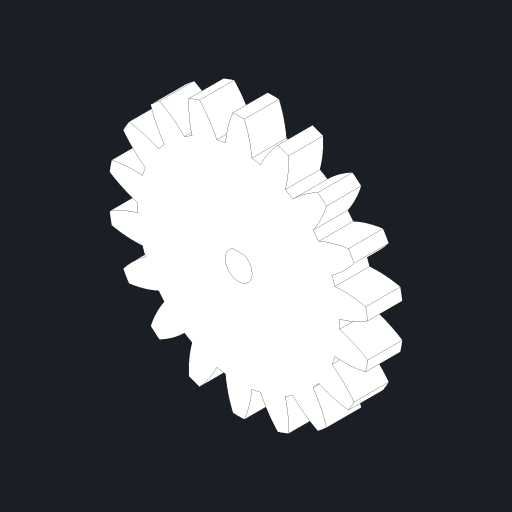
# Autodesk Inventor part: Spur Gear1
Saved by Autodesk Inventor 2024.3 (Build 283343000, 343)
## iProperties
CustomPartVersion: 1
Created: 2024-08-15
Part Number: Spur Gear1
Material: Steel
Document SubType Name: Modeling
Designer: Niler
Categories: <?xml version="1.0" encoding="UTF-16"?> <MemberInstance><Categories><FamilyTemplate><FamilyTemplateParameter ValueType="xs:double" Id="1" ObjectReferenceKey="da_z" ObjectType="kUserParameterObject"/><FamilyTemplateParameter ValueType="xs:double" Id="2" ObjectReferenceKey="da_b" ObjectType="kUserParameterObject"/><FamilyTemplateParameter ValueType="xs:double" Id="3" ObjectReferenceKey="da_beta" ObjectType="kUserParameterObject"/><FamilyTemplateParameter ValueType="xs:double" Id="4" ObjectReferenceKey="da_da" ObjectType="kUserParameterObject"/><FamilyTemplateParameter ValueType="xs:double" Id="5" ObjectReferenceKey="da_aw" ObjectType="kUserParameterObject"/><FamilyTemplateParameter ValueType="xs:string" Id="6" ObjectReferenceKey="EAIAABAAAACIAQAAAAAAAIAAAAAAAAAA" ObjectType="83910656" SubObjectId="SurfaceGeometry"/></FamilyTemplate><ParamToTemplateMap><ParamToTemplate CategoryParameter="//CategoryParameter[@InternalName='046C89C9-8512-4d59-83FE-43B91F4F132A']" TemplateParameter="1"/><ParamToTemplate CategoryParameter="//CategoryParameter[@InternalName='2552DF32-E462-4b46-AEBF-C6C7768E72AC']" TemplateParameter="2"/><ParamToTemplate CategoryParameter="//CategoryParameter[@InternalName='C9EE641D-15FC-4fae-A226-E94C4372FDD7']" TemplateParameter="3"/><ParamToTemplate><ParamToTemplate CategoryParameter="//CategoryParameter[@InternalName='00B6519A-459B-49c7-AD84-2E56D39A5744']" ConstantValue="0.000000"/></ParamToTemplate><ParamToTemplate><ParamToTemplate CategoryParameter="//CategoryParameter[@InternalName='04B31F0E-C7A6-4894-AA32-9629BEFACF47']" ConstantValue="1.000000"/></ParamToTemplate><ParamToTemplate><ParamToTemplate CategoryParameter="//CategoryParameter[@InternalName='43CBEC2E-7847-49e7-A936-2F7889FCB2D9']" ConstantValue="0.250000"/></ParamToTemplate><ParamToTemplate><ParamToTemplate CategoryParameter="//CategoryParameter[@InternalName='B1EFC894-105D-4ebd-86BF-FA20ED196853']" ConstantValue="0.350000"/></ParamToTemplate><ParamToTemplate><ParamToTemplate CategoryParameter="//CategoryParameter[@InternalName='51175063-3D10-4879-93E8-6246FE8B403D']" ConstantValue="2060000000.000000"/></ParamToTemplate><ParamToTemplate><ParamToTemplate CategoryParameter="//CategoryParameter[@InternalName='A3A52E27-4454-46a9-B0BD-C932399B70AF']" ConstantValue="0.300000"/></ParamToTemplate><ParamToTemplate><ParamToTemplate CategoryParameter="//CategoryParameter[@InternalName='91B76062-C214-41d9-B1B9-14D2AB99603D']" ConstantValue="0.300000"/></ParamToTemplate><ParamToTemplate><ParamToTemplate CategoryParameter="//CategoryParameter[@InternalName='374E806E-8B8A-4dda-A9AA-1039D6500AD2']" ConstantValue="3.333333"/></ParamToTemplate><ParamToTemplate><ParamToTemplate CategoryParameter="//CategoryParameter[@InternalName='2D373A89-B862-43d6-8D0B-0CBF12AB9F6C']" ConstantValue="0.349066"/></ParamToTemplate><ParamToTemplate CategoryParameter="//CategoryParameter[@InternalName='37777632-D6A2-4fac-9D53-DB8ACD95C989']" TemplateParameter="4"/><ParamToTemplate CategoryParameter="//CategoryParameter[@InternalName='FD1017F1-B727-4f7e-9707-0F86F1FF9423']" TemplateParameter="5"/><ParamToTemplate><ParamToTemplate CategoryParameter="//CategoryParameter[@InternalName='9E1B4470-B2D3-4ff1-B813-535BB4CDF51A']" ConstantValue="3520000.000000"/></ParamToTemplate><ParamToTemplate><ParamToTemplate CategoryParameter="//CategoryParameter[@InternalName='F8452263-BFF6-458c-9FB1-07C4B99E95CD']" ConstantValue="11400000.000000"/></ParamToTemplate><ParamToTemplate><ParamToTemplate CategoryParameter="//CategoryParameter[@InternalName='3E3BB259-FD49-497f-8171-6EBC954A3479']" ConstantValue="2.000000"/></ParamToTemplate><ParamToTemplate CategoryParameter="//CategoryParameter[@InternalName='27C3BAF2-7550-4e4b-AE2C-0DB134B7D9B7']" TemplateParameter="6"/></ParamToTemplateMap><Category DisplayName="Gear" InternalName="DC85795E-93AB-48d5-8EEE-5A27447B64BD" Mnemonic="Gear"><CategoryParameter DisplayName="z" InternalName="046C89C9-8512-4d59-83FE-43B91F4F132A" Mnemonic="z"/><CategoryParameter DisplayName="b" InternalName="2552DF32-E462-4b46-AEBF-C6C7768E72AC" Mnemonic="b"/><CategoryParameter DisplayName="||b|" InternalName="C9EE641D-15FC-4fae-A226-E94C4372FDD7" Mnemonic="beta"/><CategoryParameter DisplayName="x" InternalName="00B6519A-459B-49c7-AD84-2E56D39A5744" Mnemonic="x"/><CategoryParameter DisplayName="a*" InternalName="04B31F0E-C7A6-4894-AA32-9629BEFACF47" Mnemonic="a"/><CategoryParameter DisplayName="c*" InternalName="43CBEC2E-7847-49e7-A936-2F7889FCB2D9" Mnemonic="c"/><CategoryParameter DisplayName="r|.f|*" InternalName="B1EFC894-105D-4ebd-86BF-FA20ED196853" Mnemonic="rf"/><CategoryParameter DisplayName="E" InternalName="51175063-3D10-4879-93E8-6246FE8B403D" Mnemonic="E"/><CategoryParameter DisplayName="||m|" InternalName="A3A52E27-4454-46a9-B0BD-C932399B70AF" Mnemonic="mi"/><Category DisplayName="SpurGear" InternalName="26C5A22E-A91E-4dfd-A3B3-23CCAFAE1764" Mnemonic="SpurGear"><CategoryParameter DisplayName="m" InternalName="91B76062-C214-41d9-B1B9-14D2AB99603D" Mnemonic="m"/><CategoryParameter DisplayName="P" InternalName="374E806E-8B8A-4dda-A9AA-1039D6500AD2" Mnemonic="PP"/><CategoryParameter DisplayName="||a|" InternalName="2D373A89-B862-43d6-8D0B-0CBF12AB9F6C" Mnemonic="alpha"/><CategoryParameter DisplayName="d|.a|" InternalName="37777632-D6A2-4fac-9D53-DB8ACD95C989" Mnemonic="da"/><CategoryParameter DisplayName="a|.w|" InternalName="FD1017F1-B727-4f7e-9707-0F86F1FF9423" Mnemonic="aw"/><CategoryParameter DisplayName="||s||.Flim|" InternalName="9E1B4470-B2D3-4ff1-B813-535BB4CDF51A" Mnemonic="sFlim"/><CategoryParameter DisplayName="||s||.Hlim|" InternalName="F8452263-BFF6-458c-9FB1-07C4B99E95CD" Mnemonic="sHlim"/><CategoryParameter DisplayName="type" InternalName="3E3BB259-FD49-497f-8171-6EBC954A3479" Mnemonic="type"/><CategoryParameter DisplayName="PitchDiameter" InternalName="27C3BAF2-7550-4e4b-AE2C-0DB134B7D9B7" Mnemonic="IDS_PITCHDIAM"/></Category></Category></Categories></MemberInstance>
Density: 1 g/cm^3
Appearance: Steel
Author: Niler
Autodesk Inventor part; units mm, degrees
sketch "Sketch1" plane through (0, 0, 0) normal (0, 0, 1) x (1, 0, 0)
  circle A0 centre (0, 0) radius 30
  dimension "d0" = 60
  constraints: 1 centre point
  measures "d0" diameter of A0
extrude "Extrusion1" add sketch "Sketch1" along normal blind 8
ref_plane "Work Plane2" through (0, 0, 4) normal (0, 0, 1) x (1, 0, 0)
sketch "Sketch2" plane through (0, 0, 0) normal (0, 0, -1) x (-1, 0, 0)
  circle A0 centre (0, 0) radius 30 projected
  circle A1 centre (0, 0) radius 27
  dimension "d3" = 54
  constraints: 1 centre point, 1 coincident
  measures "d3" diameter of A1
surface extrude "Pitch Diameter" sketch "Sketch2" against normal through all shown no curves A1
ref_plane "Work Plane8" through (0, 0, 0) normal (0.9848078, 0.1736482, 0) x (0, 0, 1)
ref_plane "Work Plane9" through (0, 0, 0) normal (1, 0, 0) x (0, 1, 0)
spur gear teeth "Spur Gear" teeth 18 pitch diameter 54 tip diameter 60 root diameter 46.5 face width 8 start plane through (0, 0, 0) normal (0, 0, -1) x (-1, 0, 0)
sketch "Sketch3" plane through (0, 0, 0) normal (0, 0, -1) x (-1, 0, 0)
  circle A0 centre (0, 0) radius 3.1
  arc A1 (10.7357, 20.623) -> (11.4805, 27.7164) centre (-12.0166, 26.5979) ccw projected
  arc A2 (11.4805, 27.7164) -> (9.0212, 28.6115) centre (0, 0) ccw projected
  arc A3 (9.0212, 28.6115) -> (5.0322, 22.6989) centre (26.3021, 12.6511) ccw projected
  arc A4 (5.0322, 22.6989) -> (3.0347, 23.0511) centre (0, 0) ccw projected
  arc A5 (3.0347, 23.0511) -> (1.3086, 29.9714) centre (-20.389, 20.8839) ccw projected
  arc A6 (1.3086, 29.9714) -> (-1.3086, 29.9714) centre (0, 0) ccw projected
  arc A7 (-1.3086, 29.9714) -> (-3.0347, 23.0511) centre (20.389, 20.8839) ccw projected
  arc A8 (-3.0347, 23.0511) -> (-5.0322, 22.6989) centre (0, 0) ccw projected
  arc A9 (-5.0322, 22.6989) -> (-9.0212, 28.6115) centre (-26.3021, 12.6511) ccw projected
  arc A10 (-9.0212, 28.6115) -> (-11.4805, 27.7164) centre (0, 0) ccw projected
  arc A11 (-11.4805, 27.7164) -> (-10.7357, 20.623) centre (12.0166, 26.5979) ccw projected
  arc A12 (-10.7357, 20.623) -> (-12.4922, 19.6089) centre (0, 0) ccw projected
  arc A13 (-12.4922, 19.6089) -> (-18.2628, 23.8006) centre (-29.0428, 2.8923) ccw projected
  arc A14 (-18.2628, 23.8006) -> (-20.2677, 22.1183) centre (0, 0) ccw projected
  arc A15 (-20.2677, 22.1183) -> (-17.1417, 15.7075) centre (2.1949, 29.1038) ccw projected
  arc A16 (-17.1417, 15.7075) -> (-18.4455, 14.1537) centre (0, 0) ccw projected
  arc A17 (-18.4455, 14.1537) -> (-25.3017, 16.119) centre (-28.2805, -7.2154) ccw projected
  arc A18 (-25.3017, 16.119) -> (-26.6103, 13.8525) centre (0, 0) ccw projected
  arc A19 (-26.6103, 13.8525) -> (-21.4802, 8.8974) centre (-7.8916, 28.0993) ccw projected
  arc A20 (-21.4802, 8.8974) -> (-22.1739, 6.9914) centre (0, 0) ccw projected
  arc A21 (-22.1739, 6.9914) -> (-29.2889, 6.4932) centre (-24.1072, -16.4527) ccw projected
  arc A22 (-29.2889, 6.4932) -> (-29.7433, 3.9158) centre (0, 0) ccw projected
  arc A23 (-29.7433, 3.9158) -> (-23.2279, 1.0142) centre (-17.0262, 23.7057) ccw projected
  arc A24 (-23.2279, 1.0142) -> (-23.2279, -1.0142) centre (0, 0) ccw projected
  arc A25 (-23.2279, -1.0142) -> (-29.7433, -3.9158) centre (-17.0262, -23.7057) ccw projected
  arc A26 (-29.7433, -3.9158) -> (-29.2889, -6.4932) centre (0, 0) ccw projected
  arc A27 (-29.2889, -6.4932) -> (-22.1739, -6.9914) centre (-24.1072, 16.4527) ccw projected
  arc A28 (-22.1739, -6.9914) -> (-21.4802, -8.8974) centre (0, 0) ccw projected
  arc A29 (-21.4802, -8.8974) -> (-26.6103, -13.8525) centre (-7.8916, -28.0993) ccw projected
  arc A30 (-26.6103, -13.8525) -> (-25.3017, -16.119) centre (0, 0) ccw projected
  arc A31 (-25.3017, -16.119) -> (-18.4455, -14.1537) centre (-28.2805, 7.2154) ccw projected
  arc A32 (-18.4455, -14.1537) -> (-17.1417, -15.7075) centre (0, 0) ccw projected
  arc A33 (-17.1417, -15.7075) -> (-20.2677, -22.1183) centre (2.1949, -29.1038) ccw projected
  arc A34 (-20.2677, -22.1183) -> (-18.2628, -23.8006) centre (0, 0) ccw projected
  arc A35 (-18.2628, -23.8006) -> (-12.4922, -19.6089) centre (-29.0428, -2.8923) ccw projected
  arc A36 (-12.4922, -19.6089) -> (-10.7357, -20.623) centre (0, 0) ccw projected
  arc A37 (-10.7357, -20.623) -> (-11.4805, -27.7164) centre (12.0166, -26.5979) ccw projected
  arc A38 (-11.4805, -27.7164) -> (-9.0212, -28.6115) centre (0, 0) ccw projected
  arc A39 (-9.0212, -28.6115) -> (-5.0322, -22.6989) centre (-26.3021, -12.6511) ccw projected
  arc A40 (-5.0322, -22.6989) -> (-3.0347, -23.0511) centre (0, 0) ccw projected
  arc A41 (-3.0347, -23.0511) -> (-1.3086, -29.9714) centre (20.389, -20.8839) ccw projected
  arc A42 (-1.3086, -29.9714) -> (1.3086, -29.9714) centre (0, 0) ccw projected
  arc A43 (1.3086, -29.9714) -> (3.0347, -23.0511) centre (-20.389, -20.8839) ccw projected
  arc A44 (3.0347, -23.0511) -> (5.0322, -22.6989) centre (0, 0) ccw projected
  arc A45 (5.0322, -22.6989) -> (9.0212, -28.6115) centre (26.3021, -12.6511) ccw projected
  arc A46 (9.0212, -28.6115) -> (11.4805, -27.7164) centre (0, 0) ccw projected
  arc A47 (11.4805, -27.7164) -> (10.7357, -20.623) centre (-12.0166, -26.5979) ccw projected
  arc A48 (10.7357, -20.623) -> (12.4922, -19.6089) centre (0, 0) ccw projected
  arc A49 (12.4922, -19.6089) -> (18.2628, -23.8006) centre (29.0428, -2.8923) ccw projected
  arc A50 (18.2628, -23.8006) -> (20.2677, -22.1183) centre (0, 0) ccw projected
  arc A51 (20.2677, -22.1183) -> (17.1417, -15.7075) centre (-2.1949, -29.1038) ccw projected
  arc A52 (17.1417, -15.7075) -> (18.4455, -14.1537) centre (0, 0) ccw projected
  arc A53 (18.4455, -14.1537) -> (25.3017, -16.119) centre (28.2805, 7.2154) ccw projected
  arc A54 (25.3017, -16.119) -> (26.6103, -13.8525) centre (0, 0) ccw projected
  arc A55 (26.6103, -13.8525) -> (21.4802, -8.8974) centre (7.8916, -28.0993) ccw projected
  arc A56 (21.4802, -8.8974) -> (22.1739, -6.9914) centre (0, 0) ccw projected
  arc A57 (22.1739, -6.9914) -> (29.2889, -6.4932) centre (24.1072, 16.4527) ccw projected
  arc A58 (29.2889, -6.4932) -> (29.7433, -3.9158) centre (0, 0) ccw projected
  arc A59 (29.7433, -3.9158) -> (23.2279, -1.0142) centre (17.0262, -23.7057) ccw projected
  arc A60 (23.2279, -1.0142) -> (23.2279, 1.0142) centre (0, 0) ccw projected
  arc A61 (23.2279, 1.0142) -> (29.7433, 3.9158) centre (17.0262, 23.7057) ccw projected
  arc A62 (29.7433, 3.9158) -> (29.2889, 6.4932) centre (0, 0) ccw projected
  arc A63 (29.2889, 6.4932) -> (22.1739, 6.9914) centre (24.1072, -16.4527) ccw projected
  arc A64 (22.1739, 6.9914) -> (21.4802, 8.8974) centre (0, 0) ccw projected
  arc A65 (21.4802, 8.8974) -> (26.6103, 13.8525) centre (7.8916, 28.0993) ccw projected
  arc A66 (26.6103, 13.8525) -> (25.3017, 16.119) centre (0, 0) ccw projected
  arc A67 (25.3017, 16.119) -> (18.4455, 14.1537) centre (28.2805, -7.2154) ccw projected
  arc A68 (18.4455, 14.1537) -> (17.1417, 15.7075) centre (0, 0) ccw projected
  arc A69 (17.1417, 15.7075) -> (20.2677, 22.1183) centre (-2.1949, 29.1038) ccw projected
  arc A70 (20.2677, 22.1183) -> (18.2628, 23.8006) centre (0, 0) ccw projected
  arc A71 (18.2628, 23.8006) -> (12.4922, 19.6089) centre (29.0428, 2.8923) ccw projected
  arc A72 (12.4922, 19.6089) -> (10.7357, 20.623) centre (0, 0) ccw projected
  line L0 (-1.2707, 2.8276) -> (1.2707, 2.8276)
  dimension "d49" = 6.2
  constraints: 2 end point, 2 point on circle, 1 centre point, 1 coincident, 1 horizontal
  measures "d49" diameter of A0
extrude "Extrusion2" cut sketch "Sketch3" against normal through all contours A0 L0 picked at (-0.932, 0.7539)
equation "\"d0\" = da_da"
equation "\"d1\" = da_b"
equation "\"d3\" = da_d"
equation "\"d16\" = da_aw"
equation "\"d43\" = da_aw"
equation "\"d46\" = da_aw"
equation "\"da_da\" = 60"
equation "\"da_b\" = 8"
equation "\"da_d\" = 54"
equation "\"da_aw\" = 78"
body "Solid1"
body "Srf1"
